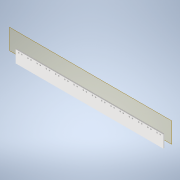
# Autodesk Inventor part: sideplate
Saved by Autodesk Inventor 2021 (Build 250183000, 183)
## iProperties
Created: 2021-04-17
Part Number: sideplate
Material: Generic
Document SubType Name: Modeling
Designer: gfellows
Density: 1 g/cm^3
Appearance: Default
Author: gfellows
Autodesk Inventor part; units mm, degrees
ref_plane "YZ Plane" through (0, 0, 0) normal (1, 0, 0) x (0, 1, 0)
ref_plane "XZ Plane" through (0, 0, 0) normal (0, 1, 0) x (-1, 0, 0)
ref_plane "XY Plane" through (0, 0, 0) normal (0, 0, 1) x (1, 0, 0)
ref_plane "Work Plane1" through (0, 0, 0) normal (0, 0, 1) x (1, 0, 0)
sketch "Sketch1" plane through (0, 0, 0) normal (0, 0, 1) x (1, 0, 0)
  line L0 (0, 0) -> (-384, 0) projected
  line L1 (-384, 0) -> (-384, -48) projected
  line L2 (0, -48) -> (-384, -48) projected
  line L3 (0, 0) -> (0, -48) projected
  line L4 (-31.0711, -33.8995) -> (-30.5858, -33.4142) projected
  arc A0 (-33.8995, -31.0711) -> (-31.0711, -33.8995) centre (-32.4853, -32.4853) ccw projected
  line L5 (-33.8995, -31.0711) -> (-33.4142, -30.5858) projected
  arc A1 (-30.5858, -33.4142) -> (-33.4142, -30.5858) centre (-32, -32) ccw projected
  circle A2 centre (-16, -40) radius 2 projected
  circle A3 centre (-32, -40) radius 2 projected
  arc A4 (-38.5858, -30.5858) -> (-41.4142, -33.4142) centre (-40, -32) ccw projected
  line L6 (-38.1005, -31.0711) -> (-38.5858, -30.5858) projected
  arc A5 (-40.9289, -33.8995) -> (-38.1005, -31.0711) centre (-39.5147, -32.4853) ccw projected
  line L7 (-40.9289, -33.8995) -> (-41.4142, -33.4142) projected
  arc A6 (-41.4142, -14.5858) -> (-38.5858, -17.4142) centre (-40, -16) ccw projected
  line L8 (-40.9289, -14.1005) -> (-41.4142, -14.5858) projected
  arc A7 (-38.1005, -16.9289) -> (-40.9289, -14.1005) centre (-39.5147, -15.5147) ccw projected
  line L9 (-38.1005, -16.9289) -> (-38.5858, -17.4142) projected
  circle A8 centre (-40, -8) radius 2 projected
  arc A9 (-9.4142, -17.4142) -> (-6.5858, -14.5858) centre (-8, -16) ccw projected
  line L10 (-9.8995, -16.9289) -> (-9.4142, -17.4142) projected
  arc A10 (-7.0711, -14.1005) -> (-9.8995, -16.9289) centre (-8.4853, -15.5147) ccw projected
  line L11 (-7.0711, -14.1005) -> (-6.5858, -14.5858) projected
  circle A11 centre (-24, -24) radius 7 projected
  line L12 (-22, -8) -> (-22, -12.6863) projected
  arc A12 (-26, -12.6863) -> (-22, -12.6863) centre (-24, -12.6863) ccw projected
  line L13 (-26, -8) -> (-26, -12.6863) projected
  arc A13 (-22, -8) -> (-26, -8) centre (-24, -8) ccw projected
  line L14 (-11.3137, -26) -> (-12.6863, -26) projected
  arc A14 (-12.6863, -22) -> (-12.6863, -26) centre (-12.6863, -24) ccw projected
  line L15 (-12.6863, -22) -> (-11.3137, -22) projected
  arc A15 (-11.3137, -26) -> (-11.3137, -22) centre (-11.3137, -24) ccw projected
  line L16 (-26, -40) -> (-26, -35.3137) projected
  arc A16 (-22, -35.3137) -> (-26, -35.3137) centre (-24, -35.3137) ccw projected
  line L17 (-22, -40) -> (-22, -35.3137) projected
  arc A17 (-26, -40) -> (-22, -40) centre (-24, -40) ccw projected
  line L18 (-36.6863, -22) -> (-35.3137, -22) projected
  arc A18 (-35.3137, -26) -> (-35.3137, -22) centre (-35.3137, -24) ccw projected
  line L19 (-35.3137, -26) -> (-36.6863, -26) projected
  arc A19 (-36.6863, -22) -> (-36.6863, -26) centre (-36.6863, -24) ccw projected
  circle A20 centre (-16, -8) radius 2 projected
  circle A21 centre (-8, -8) radius 2 projected
  arc A22 (-6.5858, -33.4142) -> (-9.4142, -30.5858) centre (-8, -32) ccw projected
  line L20 (-7.0711, -33.8995) -> (-6.5858, -33.4142) projected
  arc A23 (-9.8995, -31.0711) -> (-7.0711, -33.8995) centre (-8.4853, -32.4853) ccw projected
  line L21 (-9.8995, -31.0711) -> (-9.4142, -30.5858) projected
  circle A24 centre (-8, -40) radius 2 projected
  circle A25 centre (-32, -8) radius 2 projected
  circle A26 centre (-40, -40) radius 2 projected
  line L22 (-14.1005, -31.0711) -> (-14.5858, -30.5858) projected
  arc A27 (-16.9289, -33.8995) -> (-14.1005, -31.0711) centre (-15.5147, -32.4853) ccw projected
  line L23 (-16.9289, -33.8995) -> (-17.4142, -33.4142) projected
  arc A28 (-14.5858, -30.5858) -> (-17.4142, -33.4142) centre (-16, -32) ccw projected
  arc A29 (-17.4142, -14.5858) -> (-14.5858, -17.4142) centre (-16, -16) ccw projected
  line L24 (-16.9289, -14.1005) -> (-17.4142, -14.5858) projected
  arc A30 (-14.1005, -16.9289) -> (-16.9289, -14.1005) centre (-15.5147, -15.5147) ccw projected
  line L25 (-14.1005, -16.9289) -> (-14.5858, -17.4142) projected
  line L26 (-31.0711, -14.1005) -> (-30.5858, -14.5858) projected
  arc A31 (-33.4142, -17.4142) -> (-30.5858, -14.5858) centre (-32, -16) ccw projected
  line L27 (-33.8995, -16.9289) -> (-33.4142, -17.4142) projected
  arc A32 (-31.0711, -14.1005) -> (-33.8995, -16.9289) centre (-32.4853, -15.5147) ccw projected
  line L28 (-367.0711, -14.1005) -> (-366.5858, -14.5858) projected
  arc A33 (-369.4142, -17.4142) -> (-366.5858, -14.5858) centre (-368, -16) ccw projected
  line L29 (-369.8995, -16.9289) -> (-369.4142, -17.4142) projected
  arc A34 (-367.0711, -14.1005) -> (-369.8995, -16.9289) centre (-368.4853, -15.5147) ccw projected
  circle A35 centre (-376, -40) radius 2 projected
  circle A36 centre (-368, -8) radius 2 projected
  line L30 (-372.6863, -22) -> (-371.3137, -22) projected
  arc A37 (-371.3137, -26) -> (-371.3137, -22) centre (-371.3137, -24) ccw projected
  line L31 (-371.3137, -26) -> (-372.6863, -26) projected
  arc A38 (-372.6863, -22) -> (-372.6863, -26) centre (-372.6863, -24) ccw projected
  line L32 (-362, -40) -> (-362, -35.3137) projected
  arc A39 (-358, -35.3137) -> (-362, -35.3137) centre (-360, -35.3137) ccw projected
  line L33 (-358, -40) -> (-358, -35.3137) projected
  arc A40 (-362, -40) -> (-358, -40) centre (-360, -40) ccw projected
  line L34 (-358, -8) -> (-358, -12.6863) projected
  arc A41 (-362, -12.6863) -> (-358, -12.6863) centre (-360, -12.6863) ccw projected
  line L35 (-362, -8) -> (-362, -12.6863) projected
  arc A42 (-358, -8) -> (-362, -8) centre (-360, -8) ccw projected
  circle A43 centre (-360, -24) radius 7 projected
  circle A44 centre (-376, -8) radius 2 projected
  arc A45 (-377.4142, -14.5858) -> (-374.5858, -17.4142) centre (-376, -16) ccw projected
  line L36 (-376.9289, -14.1005) -> (-377.4142, -14.5858) projected
  arc A46 (-374.1005, -16.9289) -> (-376.9289, -14.1005) centre (-375.5147, -15.5147) ccw projected
  line L37 (-374.1005, -16.9289) -> (-374.5858, -17.4142) projected
  arc A47 (-374.5858, -30.5858) -> (-377.4142, -33.4142) centre (-376, -32) ccw projected
  line L38 (-374.1005, -31.0711) -> (-374.5858, -30.5858) projected
  arc A48 (-376.9289, -33.8995) -> (-374.1005, -31.0711) centre (-375.5147, -32.4853) ccw projected
  line L39 (-376.9289, -33.8995) -> (-377.4142, -33.4142) projected
  circle A49 centre (-368, -40) radius 2 projected
  line L40 (-367.0711, -33.8995) -> (-366.5858, -33.4142) projected
  arc A50 (-369.8995, -31.0711) -> (-367.0711, -33.8995) centre (-368.4853, -32.4853) ccw projected
  line L41 (-369.8995, -31.0711) -> (-369.4142, -30.5858) projected
  arc A51 (-366.5858, -33.4142) -> (-369.4142, -30.5858) centre (-368, -32) ccw projected
  line L42 (-343.0711, -14.1005) -> (-342.5858, -14.5858) projected
  arc A52 (-345.4142, -17.4142) -> (-342.5858, -14.5858) centre (-344, -16) ccw projected
  line L43 (-345.8995, -16.9289) -> (-345.4142, -17.4142) projected
  arc A53 (-343.0711, -14.1005) -> (-345.8995, -16.9289) centre (-344.4853, -15.5147) ccw projected
  circle A54 centre (-352, -40) radius 2 projected
  circle A55 centre (-344, -8) radius 2 projected
  line L44 (-348.6863, -22) -> (-347.3137, -22) projected
  arc A56 (-347.3137, -26) -> (-347.3137, -22) centre (-347.3137, -24) ccw projected
  line L45 (-347.3137, -26) -> (-348.6863, -26) projected
  arc A57 (-348.6863, -22) -> (-348.6863, -26) centre (-348.6863, -24) ccw projected
  line L46 (-338, -40) -> (-338, -35.3137) projected
  arc A58 (-334, -35.3137) -> (-338, -35.3137) centre (-336, -35.3137) ccw projected
  line L47 (-334, -40) -> (-334, -35.3137) projected
  arc A59 (-338, -40) -> (-334, -40) centre (-336, -40) ccw projected
  line L48 (-334, -8) -> (-334, -12.6863) projected
  arc A60 (-338, -12.6863) -> (-334, -12.6863) centre (-336, -12.6863) ccw projected
  line L49 (-338, -8) -> (-338, -12.6863) projected
  arc A61 (-334, -8) -> (-338, -8) centre (-336, -8) ccw projected
  circle A62 centre (-336, -24) radius 7 projected
  circle A63 centre (-352, -8) radius 2 projected
  arc A64 (-353.4142, -14.5858) -> (-350.5858, -17.4142) centre (-352, -16) ccw projected
  line L50 (-352.9289, -14.1005) -> (-353.4142, -14.5858) projected
  arc A65 (-350.1005, -16.9289) -> (-352.9289, -14.1005) centre (-351.5147, -15.5147) ccw projected
  line L51 (-350.1005, -16.9289) -> (-350.5858, -17.4142) projected
  arc A66 (-350.5858, -30.5858) -> (-353.4142, -33.4142) centre (-352, -32) ccw projected
  line L52 (-350.1005, -31.0711) -> (-350.5858, -30.5858) projected
  arc A67 (-352.9289, -33.8995) -> (-350.1005, -31.0711) centre (-351.5147, -32.4853) ccw projected
  line L53 (-352.9289, -33.8995) -> (-353.4142, -33.4142) projected
  circle A68 centre (-344, -40) radius 2 projected
  line L54 (-343.0711, -33.8995) -> (-342.5858, -33.4142) projected
  arc A69 (-345.8995, -31.0711) -> (-343.0711, -33.8995) centre (-344.4853, -32.4853) ccw projected
  line L55 (-345.8995, -31.0711) -> (-345.4142, -30.5858) projected
  arc A70 (-342.5858, -33.4142) -> (-345.4142, -30.5858) centre (-344, -32) ccw projected
  line L56 (-319.0711, -14.1005) -> (-318.5858, -14.5858) projected
  arc A71 (-321.4142, -17.4142) -> (-318.5858, -14.5858) centre (-320, -16) ccw projected
  line L57 (-321.8995, -16.9289) -> (-321.4142, -17.4142) projected
  arc A72 (-319.0711, -14.1005) -> (-321.8995, -16.9289) centre (-320.4853, -15.5147) ccw projected
  circle A73 centre (-328, -40) radius 2 projected
  circle A74 centre (-320, -8) radius 2 projected
  line L58 (-324.6863, -22) -> (-323.3137, -22) projected
  arc A75 (-323.3137, -26) -> (-323.3137, -22) centre (-323.3137, -24) ccw projected
  line L59 (-323.3137, -26) -> (-324.6863, -26) projected
  arc A76 (-324.6863, -22) -> (-324.6863, -26) centre (-324.6863, -24) ccw projected
  line L60 (-314, -40) -> (-314, -35.3137) projected
  arc A77 (-310, -35.3137) -> (-314, -35.3137) centre (-312, -35.3137) ccw projected
  line L61 (-310, -40) -> (-310, -35.3137) projected
  arc A78 (-314, -40) -> (-310, -40) centre (-312, -40) ccw projected
  line L62 (-310, -8) -> (-310, -12.6863) projected
  arc A79 (-314, -12.6863) -> (-310, -12.6863) centre (-312, -12.6863) ccw projected
  line L63 (-314, -8) -> (-314, -12.6863) projected
  arc A80 (-310, -8) -> (-314, -8) centre (-312, -8) ccw projected
  circle A81 centre (-312, -24) radius 7 projected
  circle A82 centre (-328, -8) radius 2 projected
  arc A83 (-329.4142, -14.5858) -> (-326.5858, -17.4142) centre (-328, -16) ccw projected
  line L64 (-328.9289, -14.1005) -> (-329.4142, -14.5858) projected
  arc A84 (-326.1005, -16.9289) -> (-328.9289, -14.1005) centre (-327.5147, -15.5147) ccw projected
  line L65 (-326.1005, -16.9289) -> (-326.5858, -17.4142) projected
  arc A85 (-326.5858, -30.5858) -> (-329.4142, -33.4142) centre (-328, -32) ccw projected
  line L66 (-326.1005, -31.0711) -> (-326.5858, -30.5858) projected
  arc A86 (-328.9289, -33.8995) -> (-326.1005, -31.0711) centre (-327.5147, -32.4853) ccw projected
  line L67 (-328.9289, -33.8995) -> (-329.4142, -33.4142) projected
  circle A87 centre (-320, -40) radius 2 projected
  line L68 (-319.0711, -33.8995) -> (-318.5858, -33.4142) projected
  arc A88 (-321.8995, -31.0711) -> (-319.0711, -33.8995) centre (-320.4853, -32.4853) ccw projected
  line L69 (-321.8995, -31.0711) -> (-321.4142, -30.5858) projected
  arc A89 (-318.5858, -33.4142) -> (-321.4142, -30.5858) centre (-320, -32) ccw projected
  line L70 (-295.0711, -14.1005) -> (-294.5858, -14.5858) projected
  arc A90 (-297.4142, -17.4142) -> (-294.5858, -14.5858) centre (-296, -16) ccw projected
  line L71 (-297.8995, -16.9289) -> (-297.4142, -17.4142) projected
  arc A91 (-295.0711, -14.1005) -> (-297.8995, -16.9289) centre (-296.4853, -15.5147) ccw projected
  circle A92 centre (-304, -40) radius 2 projected
  circle A93 centre (-296, -8) radius 2 projected
  line L72 (-300.6863, -22) -> (-299.3137, -22) projected
  arc A94 (-299.3137, -26) -> (-299.3137, -22) centre (-299.3137, -24) ccw projected
  line L73 (-299.3137, -26) -> (-300.6863, -26) projected
  arc A95 (-300.6863, -22) -> (-300.6863, -26) centre (-300.6863, -24) ccw projected
  line L74 (-290, -40) -> (-290, -35.3137) projected
  arc A96 (-286, -35.3137) -> (-290, -35.3137) centre (-288, -35.3137) ccw projected
  line L75 (-286, -40) -> (-286, -35.3137) projected
  arc A97 (-290, -40) -> (-286, -40) centre (-288, -40) ccw projected
  line L76 (-286, -8) -> (-286, -12.6863) projected
  arc A98 (-290, -12.6863) -> (-286, -12.6863) centre (-288, -12.6863) ccw projected
  line L77 (-290, -8) -> (-290, -12.6863) projected
  arc A99 (-286, -8) -> (-290, -8) centre (-288, -8) ccw projected
  circle A100 centre (-288, -24) radius 7 projected
  circle A101 centre (-304, -8) radius 2 projected
  arc A102 (-305.4142, -14.5858) -> (-302.5858, -17.4142) centre (-304, -16) ccw projected
  line L78 (-304.9289, -14.1005) -> (-305.4142, -14.5858) projected
  arc A103 (-302.1005, -16.9289) -> (-304.9289, -14.1005) centre (-303.5147, -15.5147) ccw projected
  line L79 (-302.1005, -16.9289) -> (-302.5858, -17.4142) projected
  arc A104 (-302.5858, -30.5858) -> (-305.4142, -33.4142) centre (-304, -32) ccw projected
  line L80 (-302.1005, -31.0711) -> (-302.5858, -30.5858) projected
  arc A105 (-304.9289, -33.8995) -> (-302.1005, -31.0711) centre (-303.5147, -32.4853) ccw projected
  line L81 (-304.9289, -33.8995) -> (-305.4142, -33.4142) projected
  circle A106 centre (-296, -40) radius 2 projected
  line L82 (-295.0711, -33.8995) -> (-294.5858, -33.4142) projected
  arc A107 (-297.8995, -31.0711) -> (-295.0711, -33.8995) centre (-296.4853, -32.4853) ccw projected
  line L83 (-297.8995, -31.0711) -> (-297.4142, -30.5858) projected
  arc A108 (-294.5858, -33.4142) -> (-297.4142, -30.5858) centre (-296, -32) ccw projected
  line L84 (-271.0711, -14.1005) -> (-270.5858, -14.5858) projected
  arc A109 (-273.4142, -17.4142) -> (-270.5858, -14.5858) centre (-272, -16) ccw projected
  line L85 (-273.8995, -16.9289) -> (-273.4142, -17.4142) projected
  arc A110 (-271.0711, -14.1005) -> (-273.8995, -16.9289) centre (-272.4853, -15.5147) ccw projected
  circle A111 centre (-280, -40) radius 2 projected
  circle A112 centre (-272, -8) radius 2 projected
  line L86 (-276.6863, -22) -> (-275.3137, -22) projected
  arc A113 (-275.3137, -26) -> (-275.3137, -22) centre (-275.3137, -24) ccw projected
  line L87 (-275.3137, -26) -> (-276.6863, -26) projected
  arc A114 (-276.6863, -22) -> (-276.6863, -26) centre (-276.6863, -24) ccw projected
  line L88 (-266, -40) -> (-266, -35.3137) projected
  arc A115 (-262, -35.3137) -> (-266, -35.3137) centre (-264, -35.3137) ccw projected
  line L89 (-262, -40) -> (-262, -35.3137) projected
  arc A116 (-266, -40) -> (-262, -40) centre (-264, -40) ccw projected
  line L90 (-262, -8) -> (-262, -12.6863) projected
  arc A117 (-266, -12.6863) -> (-262, -12.6863) centre (-264, -12.6863) ccw projected
  line L91 (-266, -8) -> (-266, -12.6863) projected
  arc A118 (-262, -8) -> (-266, -8) centre (-264, -8) ccw projected
  circle A119 centre (-264, -24) radius 7 projected
  circle A120 centre (-280, -8) radius 2 projected
  arc A121 (-281.4142, -14.5858) -> (-278.5858, -17.4142) centre (-280, -16) ccw projected
  line L92 (-280.9289, -14.1005) -> (-281.4142, -14.5858) projected
  arc A122 (-278.1005, -16.9289) -> (-280.9289, -14.1005) centre (-279.5147, -15.5147) ccw projected
  line L93 (-278.1005, -16.9289) -> (-278.5858, -17.4142) projected
  arc A123 (-278.5858, -30.5858) -> (-281.4142, -33.4142) centre (-280, -32) ccw projected
  line L94 (-278.1005, -31.0711) -> (-278.5858, -30.5858) projected
  arc A124 (-280.9289, -33.8995) -> (-278.1005, -31.0711) centre (-279.5147, -32.4853) ccw projected
  line L95 (-280.9289, -33.8995) -> (-281.4142, -33.4142) projected
  circle A125 centre (-272, -40) radius 2 projected
  line L96 (-271.0711, -33.8995) -> (-270.5858, -33.4142) projected
  arc A126 (-273.8995, -31.0711) -> (-271.0711, -33.8995) centre (-272.4853, -32.4853) ccw projected
  line L97 (-273.8995, -31.0711) -> (-273.4142, -30.5858) projected
  arc A127 (-270.5858, -33.4142) -> (-273.4142, -30.5858) centre (-272, -32) ccw projected
  line L98 (-247.0711, -14.1005) -> (-246.5858, -14.5858) projected
  arc A128 (-249.4142, -17.4142) -> (-246.5858, -14.5858) centre (-248, -16) ccw projected
  line L99 (-249.8995, -16.9289) -> (-249.4142, -17.4142) projected
  arc A129 (-247.0711, -14.1005) -> (-249.8995, -16.9289) centre (-248.4853, -15.5147) ccw projected
  circle A130 centre (-256, -40) radius 2 projected
  circle A131 centre (-248, -8) radius 2 projected
  line L100 (-252.6863, -22) -> (-251.3137, -22) projected
  arc A132 (-251.3137, -26) -> (-251.3137, -22) centre (-251.3137, -24) ccw projected
  line L101 (-251.3137, -26) -> (-252.6863, -26) projected
  arc A133 (-252.6863, -22) -> (-252.6863, -26) centre (-252.6863, -24) ccw projected
  line L102 (-242, -40) -> (-242, -35.3137) projected
  arc A134 (-238, -35.3137) -> (-242, -35.3137) centre (-240, -35.3137) ccw projected
  line L103 (-238, -40) -> (-238, -35.3137) projected
  arc A135 (-242, -40) -> (-238, -40) centre (-240, -40) ccw projected
  line L104 (-238, -8) -> (-238, -12.6863) projected
  arc A136 (-242, -12.6863) -> (-238, -12.6863) centre (-240, -12.6863) ccw projected
  line L105 (-242, -8) -> (-242, -12.6863) projected
  arc A137 (-238, -8) -> (-242, -8) centre (-240, -8) ccw projected
  circle A138 centre (-240, -24) radius 7 projected
  circle A139 centre (-256, -8) radius 2 projected
  arc A140 (-257.4142, -14.5858) -> (-254.5858, -17.4142) centre (-256, -16) ccw projected
  line L106 (-256.9289, -14.1005) -> (-257.4142, -14.5858) projected
  arc A141 (-254.1005, -16.9289) -> (-256.9289, -14.1005) centre (-255.5147, -15.5147) ccw projected
  line L107 (-254.1005, -16.9289) -> (-254.5858, -17.4142) projected
  arc A142 (-254.5858, -30.5858) -> (-257.4142, -33.4142) centre (-256, -32) ccw projected
  line L108 (-254.1005, -31.0711) -> (-254.5858, -30.5858) projected
  arc A143 (-256.9289, -33.8995) -> (-254.1005, -31.0711) centre (-255.5147, -32.4853) ccw projected
  line L109 (-256.9289, -33.8995) -> (-257.4142, -33.4142) projected
  circle A144 centre (-248, -40) radius 2 projected
  line L110 (-247.0711, -33.8995) -> (-246.5858, -33.4142) projected
  arc A145 (-249.8995, -31.0711) -> (-247.0711, -33.8995) centre (-248.4853, -32.4853) ccw projected
  line L111 (-249.8995, -31.0711) -> (-249.4142, -30.5858) projected
  arc A146 (-246.5858, -33.4142) -> (-249.4142, -30.5858) centre (-248, -32) ccw projected
  line L112 (-223.0711, -14.1005) -> (-222.5858, -14.5858) projected
  arc A147 (-225.4142, -17.4142) -> (-222.5858, -14.5858) centre (-224, -16) ccw projected
  line L113 (-225.8995, -16.9289) -> (-225.4142, -17.4142) projected
  arc A148 (-223.0711, -14.1005) -> (-225.8995, -16.9289) centre (-224.4853, -15.5147) ccw projected
  circle A149 centre (-232, -40) radius 2 projected
  circle A150 centre (-224, -8) radius 2 projected
  line L114 (-228.6863, -22) -> (-227.3137, -22) projected
  arc A151 (-227.3137, -26) -> (-227.3137, -22) centre (-227.3137, -24) ccw projected
  line L115 (-227.3137, -26) -> (-228.6863, -26) projected
  arc A152 (-228.6863, -22) -> (-228.6863, -26) centre (-228.6863, -24) ccw projected
  line L116 (-218, -40) -> (-218, -35.3137) projected
  arc A153 (-214, -35.3137) -> (-218, -35.3137) centre (-216, -35.3137) ccw projected
  line L117 (-214, -40) -> (-214, -35.3137) projected
  arc A154 (-218, -40) -> (-214, -40) centre (-216, -40) ccw projected
  line L118 (-214, -8) -> (-214, -12.6863) projected
  arc A155 (-218, -12.6863) -> (-214, -12.6863) centre (-216, -12.6863) ccw projected
  line L119 (-218, -8) -> (-218, -12.6863) projected
  arc A156 (-214, -8) -> (-218, -8) centre (-216, -8) ccw projected
  circle A157 centre (-216, -24) radius 7 projected
  circle A158 centre (-232, -8) radius 2 projected
  arc A159 (-233.4142, -14.5858) -> (-230.5858, -17.4142) centre (-232, -16) ccw projected
  line L120 (-232.9289, -14.1005) -> (-233.4142, -14.5858) projected
  arc A160 (-230.1005, -16.9289) -> (-232.9289, -14.1005) centre (-231.5147, -15.5147) ccw projected
  line L121 (-230.1005, -16.9289) -> (-230.5858, -17.4142) projected
  arc A161 (-230.5858, -30.5858) -> (-233.4142, -33.4142) centre (-232, -32) ccw projected
  line L122 (-230.1005, -31.0711) -> (-230.5858, -30.5858) projected
  arc A162 (-232.9289, -33.8995) -> (-230.1005, -31.0711) centre (-231.5147, -32.4853) ccw projected
  line L123 (-232.9289, -33.8995) -> (-233.4142, -33.4142) projected
  circle A163 centre (-224, -40) radius 2 projected
  line L124 (-223.0711, -33.8995) -> (-222.5858, -33.4142) projected
  arc A164 (-225.8995, -31.0711) -> (-223.0711, -33.8995) centre (-224.4853, -32.4853) ccw projected
  line L125 (-225.8995, -31.0711) -> (-225.4142, -30.5858) projected
  arc A165 (-222.5858, -33.4142) -> (-225.4142, -30.5858) centre (-224, -32) ccw projected
  line L126 (-199.0711, -14.1005) -> (-198.5858, -14.5858) projected
  arc A166 (-201.4142, -17.4142) -> (-198.5858, -14.5858) centre (-200, -16) ccw projected
  line L127 (-201.8995, -16.9289) -> (-201.4142, -17.4142) projected
  arc A167 (-199.0711, -14.1005) -> (-201.8995, -16.9289) centre (-200.4853, -15.5147) ccw projected
  circle A168 centre (-208, -40) radius 2 projected
  circle A169 centre (-200, -8) radius 2 projected
  line L128 (-204.6863, -22) -> (-203.3137, -22) projected
  arc A170 (-203.3137, -26) -> (-203.3137, -22) centre (-203.3137, -24) ccw projected
  line L129 (-203.3137, -26) -> (-204.6863, -26) projected
  arc A171 (-204.6863, -22) -> (-204.6863, -26) centre (-204.6863, -24) ccw projected
  line L130 (-194, -40) -> (-194, -35.3137) projected
  arc A172 (-190, -35.3137) -> (-194, -35.3137) centre (-192, -35.3137) ccw projected
  line L131 (-190, -40) -> (-190, -35.3137) projected
  arc A173 (-194, -40) -> (-190, -40) centre (-192, -40) ccw projected
  line L132 (-190, -8) -> (-190, -12.6863) projected
  arc A174 (-194, -12.6863) -> (-190, -12.6863) centre (-192, -12.6863) ccw projected
  line L133 (-194, -8) -> (-194, -12.6863) projected
  arc A175 (-190, -8) -> (-194, -8) centre (-192, -8) ccw projected
  circle A176 centre (-192, -24) radius 7 projected
  circle A177 centre (-208, -8) radius 2 projected
  arc A178 (-209.4142, -14.5858) -> (-206.5858, -17.4142) centre (-208, -16) ccw projected
  line L134 (-208.9289, -14.1005) -> (-209.4142, -14.5858) projected
  arc A179 (-206.1005, -16.9289) -> (-208.9289, -14.1005) centre (-207.5147, -15.5147) ccw projected
  line L135 (-206.1005, -16.9289) -> (-206.5858, -17.4142) projected
  arc A180 (-206.5858, -30.5858) -> (-209.4142, -33.4142) centre (-208, -32) ccw projected
  line L136 (-206.1005, -31.0711) -> (-206.5858, -30.5858) projected
  arc A181 (-208.9289, -33.8995) -> (-206.1005, -31.0711) centre (-207.5147, -32.4853) ccw projected
  line L137 (-208.9289, -33.8995) -> (-209.4142, -33.4142) projected
  circle A182 centre (-200, -40) radius 2 projected
  line L138 (-199.0711, -33.8995) -> (-198.5858, -33.4142) projected
  arc A183 (-201.8995, -31.0711) -> (-199.0711, -33.8995) centre (-200.4853, -32.4853) ccw projected
  line L139 (-201.8995, -31.0711) -> (-201.4142, -30.5858) projected
  arc A184 (-198.5858, -33.4142) -> (-201.4142, -30.5858) centre (-200, -32) ccw projected
  line L140 (-175.0711, -14.1005) -> (-174.5858, -14.5858) projected
  arc A185 (-177.4142, -17.4142) -> (-174.5858, -14.5858) centre (-176, -16) ccw projected
  line L141 (-177.8995, -16.9289) -> (-177.4142, -17.4142) projected
  arc A186 (-175.0711, -14.1005) -> (-177.8995, -16.9289) centre (-176.4853, -15.5147) ccw projected
  circle A187 centre (-184, -40) radius 2 projected
  circle A188 centre (-176, -8) radius 2 projected
  line L142 (-180.6863, -22) -> (-179.3137, -22) projected
  arc A189 (-179.3137, -26) -> (-179.3137, -22) centre (-179.3137, -24) ccw projected
  line L143 (-179.3137, -26) -> (-180.6863, -26) projected
  arc A190 (-180.6863, -22) -> (-180.6863, -26) centre (-180.6863, -24) ccw projected
  line L144 (-170, -40) -> (-170, -35.3137) projected
  arc A191 (-166, -35.3137) -> (-170, -35.3137) centre (-168, -35.3137) ccw projected
  line L145 (-166, -40) -> (-166, -35.3137) projected
  arc A192 (-170, -40) -> (-166, -40) centre (-168, -40) ccw projected
  line L146 (-166, -8) -> (-166, -12.6863) projected
  arc A193 (-170, -12.6863) -> (-166, -12.6863) centre (-168, -12.6863) ccw projected
  line L147 (-170, -8) -> (-170, -12.6863) projected
  arc A194 (-166, -8) -> (-170, -8) centre (-168, -8) ccw projected
  circle A195 centre (-168, -24) radius 7 projected
  circle A196 centre (-184, -8) radius 2 projected
  arc A197 (-185.4142, -14.5858) -> (-182.5858, -17.4142) centre (-184, -16) ccw projected
  line L148 (-184.9289, -14.1005) -> (-185.4142, -14.5858) projected
  arc A198 (-182.1005, -16.9289) -> (-184.9289, -14.1005) centre (-183.5147, -15.5147) ccw projected
  line L149 (-182.1005, -16.9289) -> (-182.5858, -17.4142) projected
  arc A199 (-182.5858, -30.5858) -> (-185.4142, -33.4142) centre (-184, -32) ccw projected
  line L150 (-182.1005, -31.0711) -> (-182.5858, -30.5858) projected
  arc A200 (-184.9289, -33.8995) -> (-182.1005, -31.0711) centre (-183.5147, -32.4853) ccw projected
  line L151 (-184.9289, -33.8995) -> (-185.4142, -33.4142) projected
  circle A201 centre (-176, -40) radius 2 projected
  line L152 (-175.0711, -33.8995) -> (-174.5858, -33.4142) projected
  arc A202 (-177.8995, -31.0711) -> (-175.0711, -33.8995) centre (-176.4853, -32.4853) ccw projected
  line L153 (-177.8995, -31.0711) -> (-177.4142, -30.5858) projected
  arc A203 (-174.5858, -33.4142) -> (-177.4142, -30.5858) centre (-176, -32) ccw projected
  line L154 (-151.0711, -14.1005) -> (-150.5858, -14.5858) projected
  arc A204 (-153.4142, -17.4142) -> (-150.5858, -14.5858) centre (-152, -16) ccw projected
  line L155 (-153.8995, -16.9289) -> (-153.4142, -17.4142) projected
  arc A205 (-151.0711, -14.1005) -> (-153.8995, -16.9289) centre (-152.4853, -15.5147) ccw projected
  circle A206 centre (-160, -40) radius 2 projected
  circle A207 centre (-152, -8) radius 2 projected
  line L156 (-156.6863, -22) -> (-155.3137, -22) projected
  arc A208 (-155.3137, -26) -> (-155.3137, -22) centre (-155.3137, -24) ccw projected
  line L157 (-155.3137, -26) -> (-156.6863, -26) projected
  arc A209 (-156.6863, -22) -> (-156.6863, -26) centre (-156.6863, -24) ccw projected
  line L158 (-146, -40) -> (-146, -35.3137) projected
  arc A210 (-142, -35.3137) -> (-146, -35.3137) centre (-144, -35.3137) ccw projected
  line L159 (-142, -40) -> (-142, -35.3137) projected
  arc A211 (-146, -40) -> (-142, -40) centre (-144, -40) ccw projected
  line L160 (-142, -8) -> (-142, -12.6863) projected
  arc A212 (-146, -12.6863) -> (-142, -12.6863) centre (-144, -12.6863) ccw projected
  line L161 (-146, -8) -> (-146, -12.6863) projected
  arc A213 (-142, -8) -> (-146, -8) centre (-144, -8) ccw projected
  circle A214 centre (-144, -24) radius 7 projected
  circle A215 centre (-160, -8) radius 2 projected
  arc A216 (-161.4142, -14.5858) -> (-158.5858, -17.4142) centre (-160, -16) ccw projected
  line L162 (-160.9289, -14.1005) -> (-161.4142, -14.5858) projected
  arc A217 (-158.1005, -16.9289) -> (-160.9289, -14.1005) centre (-159.5147, -15.5147) ccw projected
  line L163 (-158.1005, -16.9289) -> (-158.5858, -17.4142) projected
  arc A218 (-158.5858, -30.5858) -> (-161.4142, -33.4142) centre (-160, -32) ccw projected
  line L164 (-158.1005, -31.0711) -> (-158.5858, -30.5858) projected
  arc A219 (-160.9289, -33.8995) -> (-158.1005, -31.0711) centre (-159.5147, -32.4853) ccw projected
  line L165 (-160.9289, -33.8995) -> (-161.4142, -33.4142) projected
  circle A220 centre (-152, -40) radius 2 projected
  line L166 (-151.0711, -33.8995) -> (-150.5858, -33.4142) projected
  arc A221 (-153.8995, -31.0711) -> (-151.0711, -33.8995) centre (-152.4853, -32.4853) ccw projected
  line L167 (-153.8995, -31.0711) -> (-153.4142, -30.5858) projected
  arc A222 (-150.5858, -33.4142) -> (-153.4142, -30.5858) centre (-152, -32) ccw projected
  line L168 (-127.0711, -14.1005) -> (-126.5858, -14.5858) projected
  arc A223 (-129.4142, -17.4142) -> (-126.5858, -14.5858) centre (-128, -16) ccw projected
  line L169 (-129.8995, -16.9289) -> (-129.4142, -17.4142) projected
  arc A224 (-127.0711, -14.1005) -> (-129.8995, -16.9289) centre (-128.4853, -15.5147) ccw projected
  circle A225 centre (-136, -40) radius 2 projected
  circle A226 centre (-128, -8) radius 2 projected
  line L170 (-132.6863, -22) -> (-131.3137, -22) projected
  arc A227 (-131.3137, -26) -> (-131.3137, -22) centre (-131.3137, -24) ccw projected
  line L171 (-131.3137, -26) -> (-132.6863, -26) projected
  arc A228 (-132.6863, -22) -> (-132.6863, -26) centre (-132.6863, -24) ccw projected
  line L172 (-122, -40) -> (-122, -35.3137) projected
  arc A229 (-118, -35.3137) -> (-122, -35.3137) centre (-120, -35.3137) ccw projected
  line L173 (-118, -40) -> (-118, -35.3137) projected
  arc A230 (-122, -40) -> (-118, -40) centre (-120, -40) ccw projected
  line L174 (-118, -8) -> (-118, -12.6863) projected
  arc A231 (-122, -12.6863) -> (-118, -12.6863) centre (-120, -12.6863) ccw projected
  line L175 (-122, -8) -> (-122, -12.6863) projected
  arc A232 (-118, -8) -> (-122, -8) centre (-120, -8) ccw projected
  circle A233 centre (-120, -24) radius 7 projected
  circle A234 centre (-136, -8) radius 2 projected
  arc A235 (-137.4142, -14.5858) -> (-134.5858, -17.4142) centre (-136, -16) ccw projected
  line L176 (-136.9289, -14.1005) -> (-137.4142, -14.5858) projected
  arc A236 (-134.1005, -16.9289) -> (-136.9289, -14.1005) centre (-135.5147, -15.5147) ccw projected
  line L177 (-134.1005, -16.9289) -> (-134.5858, -17.4142) projected
  arc A237 (-134.5858, -30.5858) -> (-137.4142, -33.4142) centre (-136, -32) ccw projected
  line L178 (-134.1005, -31.0711) -> (-134.5858, -30.5858) projected
  arc A238 (-136.9289, -33.8995) -> (-134.1005, -31.0711) centre (-135.5147, -32.4853) ccw projected
  line L179 (-136.9289, -33.8995) -> (-137.4142, -33.4142) projected
  circle A239 centre (-128, -40) radius 2 projected
  line L180 (-127.0711, -33.8995) -> (-126.5858, -33.4142) projected
  arc A240 (-129.8995, -31.0711) -> (-127.0711, -33.8995) centre (-128.4853, -32.4853) ccw projected
  line L181 (-129.8995, -31.0711) -> (-129.4142, -30.5858) projected
  arc A241 (-126.5858, -33.4142) -> (-129.4142, -30.5858) centre (-128, -32) ccw projected
  line L182 (-103.0711, -14.1005) -> (-102.5858, -14.5858) projected
  arc A242 (-105.4142, -17.4142) -> (-102.5858, -14.5858) centre (-104, -16) ccw projected
  line L183 (-105.8995, -16.9289) -> (-105.4142, -17.4142) projected
  arc A243 (-103.0711, -14.1005) -> (-105.8995, -16.9289) centre (-104.4853, -15.5147) ccw projected
  circle A244 centre (-112, -40) radius 2 projected
  circle A245 centre (-104, -8) radius 2 projected
  line L184 (-108.6863, -22) -> (-107.3137, -22) projected
  arc A246 (-107.3137, -26) -> (-107.3137, -22) centre (-107.3137, -24) ccw projected
  line L185 (-107.3137, -26) -> (-108.6863, -26) projected
  arc A247 (-108.6863, -22) -> (-108.6863, -26) centre (-108.6863, -24) ccw projected
  line L186 (-98, -40) -> (-98, -35.3137) projected
  arc A248 (-94, -35.3137) -> (-98, -35.3137) centre (-96, -35.3137) ccw projected
  line L187 (-94, -40) -> (-94, -35.3137) projected
  arc A249 (-98, -40) -> (-94, -40) centre (-96, -40) ccw projected
  line L188 (-94, -8) -> (-94, -12.6863) projected
  arc A250 (-98, -12.6863) -> (-94, -12.6863) centre (-96, -12.6863) ccw projected
  line L189 (-98, -8) -> (-98, -12.6863) projected
  arc A251 (-94, -8) -> (-98, -8) centre (-96, -8) ccw projected
  circle A252 centre (-96, -24) radius 7 projected
  circle A253 centre (-112, -8) radius 2 projected
  arc A254 (-113.4142, -14.5858) -> (-110.5858, -17.4142) centre (-112, -16) ccw projected
  line L190 (-112.9289, -14.1005) -> (-113.4142, -14.5858) projected
  arc A255 (-110.1005, -16.9289) -> (-112.9289, -14.1005) centre (-111.5147, -15.5147) ccw projected
  line L191 (-110.1005, -16.9289) -> (-110.5858, -17.4142) projected
  arc A256 (-110.5858, -30.5858) -> (-113.4142, -33.4142) centre (-112, -32) ccw projected
  line L192 (-110.1005, -31.0711) -> (-110.5858, -30.5858) projected
  arc A257 (-112.9289, -33.8995) -> (-110.1005, -31.0711) centre (-111.5147, -32.4853) ccw projected
  line L193 (-112.9289, -33.8995) -> (-113.4142, -33.4142) projected
  circle A258 centre (-104, -40) radius 2 projected
  line L194 (-103.0711, -33.8995) -> (-102.5858, -33.4142) projected
  arc A259 (-105.8995, -31.0711) -> (-103.0711, -33.8995) centre (-104.4853, -32.4853) ccw projected
  line L195 (-105.8995, -31.0711) -> (-105.4142, -30.5858) projected
  arc A260 (-102.5858, -33.4142) -> (-105.4142, -30.5858) centre (-104, -32) ccw projected
  line L196 (-79.0711, -14.1005) -> (-78.5858, -14.5858) projected
  arc A261 (-81.4142, -17.4142) -> (-78.5858, -14.5858) centre (-80, -16) ccw projected
  line L197 (-81.8995, -16.9289) -> (-81.4142, -17.4142) projected
  arc A262 (-79.0711, -14.1005) -> (-81.8995, -16.9289) centre (-80.4853, -15.5147) ccw projected
  circle A263 centre (-88, -40) radius 2 projected
  circle A264 centre (-80, -8) radius 2 projected
  line L198 (-84.6863, -22) -> (-83.3137, -22) projected
  arc A265 (-83.3137, -26) -> (-83.3137, -22) centre (-83.3137, -24) ccw projected
  line L199 (-83.3137, -26) -> (-84.6863, -26) projected
  arc A266 (-84.6863, -22) -> (-84.6863, -26) centre (-84.6863, -24) ccw projected
  line L200 (-74, -40) -> (-74, -35.3137) projected
  arc A267 (-70, -35.3137) -> (-74, -35.3137) centre (-72, -35.3137) ccw projected
  line L201 (-70, -40) -> (-70, -35.3137) projected
  arc A268 (-74, -40) -> (-70, -40) centre (-72, -40) ccw projected
  line L202 (-70, -8) -> (-70, -12.6863) projected
  arc A269 (-74, -12.6863) -> (-70, -12.6863) centre (-72, -12.6863) ccw projected
  line L203 (-74, -8) -> (-74, -12.6863) projected
  arc A270 (-70, -8) -> (-74, -8) centre (-72, -8) ccw projected
  circle A271 centre (-72, -24) radius 7 projected
  circle A272 centre (-88, -8) radius 2 projected
  arc A273 (-89.4142, -14.5858) -> (-86.5858, -17.4142) centre (-88, -16) ccw projected
  line L204 (-88.9289, -14.1005) -> (-89.4142, -14.5858) projected
  arc A274 (-86.1005, -16.9289) -> (-88.9289, -14.1005) centre (-87.5147, -15.5147) ccw projected
  line L205 (-86.1005, -16.9289) -> (-86.5858, -17.4142) projected
  arc A275 (-86.5858, -30.5858) -> (-89.4142, -33.4142) centre (-88, -32) ccw projected
  line L206 (-86.1005, -31.0711) -> (-86.5858, -30.5858) projected
  arc A276 (-88.9289, -33.8995) -> (-86.1005, -31.0711) centre (-87.5147, -32.4853) ccw projected
  line L207 (-88.9289, -33.8995) -> (-89.4142, -33.4142) projected
  circle A277 centre (-80, -40) radius 2 projected
  line L208 (-79.0711, -33.8995) -> (-78.5858, -33.4142) projected
  arc A278 (-81.8995, -31.0711) -> (-79.0711, -33.8995) centre (-80.4853, -32.4853) ccw projected
  line L209 (-81.8995, -31.0711) -> (-81.4142, -30.5858) projected
  arc A279 (-78.5858, -33.4142) -> (-81.4142, -30.5858) centre (-80, -32) ccw projected
  line L210 (-55.0711, -14.1005) -> (-54.5858, -14.5858) projected
  arc A280 (-57.4142, -17.4142) -> (-54.5858, -14.5858) centre (-56, -16) ccw projected
  line L211 (-57.8995, -16.9289) -> (-57.4142, -17.4142) projected
  arc A281 (-55.0711, -14.1005) -> (-57.8995, -16.9289) centre (-56.4853, -15.5147) ccw projected
  circle A282 centre (-64, -40) radius 2 projected
  circle A283 centre (-56, -8) radius 2 projected
  line L212 (-60.6863, -22) -> (-59.3137, -22) projected
  arc A284 (-59.3137, -26) -> (-59.3137, -22) centre (-59.3137, -24) ccw projected
  line L213 (-59.3137, -26) -> (-60.6863, -26) projected
  arc A285 (-60.6863, -22) -> (-60.6863, -26) centre (-60.6863, -24) ccw projected
  line L214 (-50, -40) -> (-50, -35.3137) projected
  arc A286 (-46, -35.3137) -> (-50, -35.3137) centre (-48, -35.3137) ccw projected
  line L215 (-46, -40) -> (-46, -35.3137) projected
  arc A287 (-50, -40) -> (-46, -40) centre (-48, -40) ccw projected
  line L216 (-46, -8) -> (-46, -12.6863) projected
  arc A288 (-50, -12.6863) -> (-46, -12.6863) centre (-48, -12.6863) ccw projected
  line L217 (-50, -8) -> (-50, -12.6863) projected
  arc A289 (-46, -8) -> (-50, -8) centre (-48, -8) ccw projected
  circle A290 centre (-48, -24) radius 7 projected
  circle A291 centre (-64, -8) radius 2 projected
  arc A292 (-65.4142, -14.5858) -> (-62.5858, -17.4142) centre (-64, -16) ccw projected
  line L218 (-64.9289, -14.1005) -> (-65.4142, -14.5858) projected
  arc A293 (-62.1005, -16.9289) -> (-64.9289, -14.1005) centre (-63.5147, -15.5147) ccw projected
  line L219 (-62.1005, -16.9289) -> (-62.5858, -17.4142) projected
  arc A294 (-62.5858, -30.5858) -> (-65.4142, -33.4142) centre (-64, -32) ccw projected
  line L220 (-62.1005, -31.0711) -> (-62.5858, -30.5858) projected
  arc A295 (-64.9289, -33.8995) -> (-62.1005, -31.0711) centre (-63.5147, -32.4853) ccw projected
  line L221 (-64.9289, -33.8995) -> (-65.4142, -33.4142) projected
  circle A296 centre (-56, -40) radius 2 projected
  line L222 (-55.0711, -33.8995) -> (-54.5858, -33.4142) projected
  arc A297 (-57.8995, -31.0711) -> (-55.0711, -33.8995) centre (-56.4853, -32.4853) ccw projected
  line L223 (-57.8995, -31.0711) -> (-57.4142, -30.5858) projected
  arc A298 (-54.5858, -33.4142) -> (-57.4142, -30.5858) centre (-56, -32) ccw projected
  line L224 (-384, -36) -> (0, -36)
  line L225 (0, -36) -> (0, -68)
  line L226 (0, -68) -> (-384, -68)
  line L227 (-384, -68) -> (-384, -36)
  point P0 (0, -36)
  dimension "d0" = 20
  dimension "d1" = 4
  constraints: 8 end point, 2 parallel, 2 point on line, 1 horizontal, 1 perpendicular
  measures "d0" distance between parallel lines of L226 L2
  measures "d1" distance from line of A24.centre L224
extrude "Extrusion1" add sketch "Sketch1" along normal blind 3.175 contours L3 L2 L1 L224 L32 A40 L33 L46 A59 L47 L60 A78 L61 L74 A97 L75 L88 A116 L89 L102 A135 L103 L116 A154 L117 L130 A173 L131 L144 A192 L145 L158 A211 L159 L172 A230 L173 L186 A249 L187 L200 A268 L201 L214 A287 L215 L16 A17 L17 | L225 L226 L227 L2 | L17 A17 L16 L224 | L224 L33 A40 L32 | L215 A287 L214 L224 | L224 L47 A59 L46 | L201 A268 L200 L224 | L224 L61 A78 L60 | L187 A249 L186 L224 | L224 L75 A97 L74 | L173 A230 L172 L224 | L224 L89 A116 L88 | L159 A211 L158 L224 | L224 L103 A135 L102 | L145 A192 L144 L224 | L224 L117 A154 L116 | L131 A173 L130 L224
body "Solid1"
